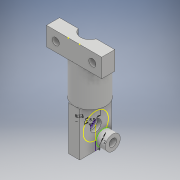
# Autodesk Inventor part: frontChassis
Saved by Autodesk Inventor 2018 (Build 220112000, 112)
## iProperties
Created: 2018-02-04
Part Number: frontChassis
Material: Generic
Document SubType Name: Modeling
Designer: Prakash
Density: 1 g/cm^3
Appearance: Default
Author: Prakash
Autodesk Inventor part; units mm, degrees
ref_plane "YZ Plane" through (0, 0, 0) normal (1, 0, 0) x (0, 1, 0)
ref_plane "XZ Plane" through (0, 0, 0) normal (0, 1, 0) x (-1, 0, 0)
ref_plane "XY Plane" through (0, 0, 0) normal (0, 0, 1) x (1, 0, 0)
sketch "Sketch1" plane through (0, 0, 0) normal (0, 0, 1) x (1, 0, 0)
  line L0 (0, 0) -> (0, 7)
  line L1 (0, 7) -> (10, 7)
  arc A0 (10, 7) -> (19.5394, 7) centre (14.7697, 8.5) ccw
  line L2 (19.5394, 7) -> (29.5394, 7)
  line L3 (29.5394, 7) -> (29.5394, 0)
  line L4 (29.5394, 0) -> (0, 0)
  dimension "d0" = 10
  dimension "d1" = 5
  dimension "d2" = 7
  dimension "d4" = 1.5
  constraints: 10 end point, 3 perpendicular, 2 collinear, 2 point on circle, 1 centre point, 1 horizontal, 1 vertical
  measures "d0" distance of L0.end L1.end
  measures "d1" radius of A0
  measures "d2" distance of L0.start L0.end
  measures "d4" distance from line of L1 A0.centre
extrude "Extrusion1" add sketch "Sketch1" against normal blind 10
sketch "Sketch3" plane through (0, 0, -10) normal (0, 0, -1) x (-1, 0, 0)
  line L0 (0, 0) -> (0, 7) projected
  line L1 (0, 7) -> (-10, 7) projected
  arc A0 (-19.5394, 7) -> (-10, 7) centre (-14.7697, 8.5) ccw projected
  line L2 (-19.5394, 7) -> (-29.5394, 7) projected
  line L3 (-29.5394, 7) -> (-29.5394, 0) projected
  line L4 (-29.5394, 0) -> (0, 0) projected
  circle A1 centre (-14.7697, 8.5) radius 5
  circle A2 centre (-14.7697, 8.5) radius 8.5
  line L5 (-29.5394, 0) -> (0, 0) projected
  constraints: 2 centre point, 1 coincident, 1 concentric, 1 tangent
extrude "Extrusion2" add sketch "Sketch3" along normal blind 20 contours A2 L2 A0 L1 | L1 A1 L2 A2
sketch "Sketch4" plane through (14.7697, 8.5, -30) normal (0, 0, -1) x (-1, 0, 0)
  line L0 (-14.7697, -8.5) -> (14.7697, -8.5) projected
  line L1 (0, -8.5) -> (3, -8.5)
  line L2 (0, -8.5) -> (-3, -8.5)
  circle A0 centre (0, 0) radius 5 projected
  circle A1 centre (0, 0) radius 8.5 projected
  line L3 (-3, -8.5) -> (3, -8.5)
  line L4 (3, -8.5) -> (3, 8.5)
  line L5 (3, 8.5) -> (-3, 8.5)
  line L6 (-3, 8.5) -> (-3, -8.5)
  dimension "d18" = 3
  dimension "d19" = 3
  constraints: 12 end point, 2 parallel, 2 point on line, 1 horizontal, 1 midpoint, 1 perpendicular, 1 tangent
  measures "d18" distance of L1.start L1.end
  measures "d19" distance of L1.start L2.end
extrude "Extrusion3" add sketch "Sketch4" along normal blind 23.5 contours L6 A1 L0 | A1 L4 L0 | A1 L6 A0 L4 | L6 L5 A1 | A1 L4 A0 L6 | L6 A0 L4 | L5 L4 A1
sketch "Sketch6" plane through (11.7697, 4.5, -30) normal (-1, 0, 0) x (0, 0, 1)
  line L0 (0, 12.5) -> (-23.5, 12.5) projected
  line L1 (-11.75, 12.5) -> (-11.75, 4)
  line L2 (-11.75, 4) -> (-23.5, 4)
  circle A0 centre (-11.75, 4) radius 6.75
  circle A1 centre (-11.75, 4) radius 3
  circle A2 centre (-11.75, 4) radius 6
  point P0 (30, -4.5)
  dimension "d26" = 8.5
  dimension "d27" = 13.5
  dimension "d28" = 6
  dimension "d29" = 12
  constraints: 4 end point, 3 centre point, 3 coincident, 1 midpoint, 1 perpendicular, 1 vertical
  measures "d26" distance of L1.start L1.end
  measures "d27" diameter of A0
  measures "d28" diameter of A1
  measures "d29" diameter of A2
extrude "Extrusion4" cut sketch "Sketch6" against normal blind 1 contours A0 L2 A2 L1 | L1 A2 L2 A0
extrude "Extrusion5" cut sketch "Sketch6" against normal blind 4 contours A2 L2 A1 L1 | L1 A1 L2 A2
extrude "Extrusion6" cut sketch "Sketch6" against normal up to surface (6 mm away) contours A1 L2 L1 | L1 L2 A1
sketch "Sketch7" plane through (17.7697, 4.5, -30) normal (1, 0, 0) x (0, 0, -1)
  line L0 (11.75, 4) -> (23.5, 4) projected
  circle A0 centre (11.75, 4) radius 6.75 projected
  line L1 (18.5, 4) -> (23.5, 4)
  circle A1 centre (19.2602, 8.1796) radius 2
  circle A2 centre (19.2602, 8.1796) radius 4
  point P0 (-30, -4.5)
  dimension "d40" = 4
  dimension "d41" = 2
  constraints: 2 centre point, 2 end point, 1 coincident, 1 collinear, 1 horizontal alignment, 1 point on line, 1 other
  measures "d40" diameter of A1
  measures "d41" radial gap between concentric circles of A1 A2
extrude "Extrusion7" add sketch "Sketch7" along normal blind 5 contours A2 A0 A1 | A0 A1 A2
extrude "Extrusion8" cut sketch "Sketch7" against normal blind 2 contours A1 A0 | A0 A1
sketch "Sketch8" plane through (0, 7, 0) normal (0, 1, 0) x (1, 0, 0)
  line L0 (0, 0) -> (10, 0) projected
  line L1 (5, 0) -> (5, 10)
  line L2 (0, 10) -> (6.4031, 10) projected
  line L3 (19.5394, 0) -> (29.5394, 0) projected
  line L4 (24.5394, 0) -> (24.5394, 10)
  point P0 (24.5394, 5)
  point P1 (5, 5)
  constraints: 4 end point, 4 midpoint, 2 vertical, 1 point on line
hole "Hole2" at (5, 7, -5) at (24.5394, 7, -5) direction (0, -1, 0) diameter 3.797 end through all clearance for "Flat Head Machine Screw (82)" size "#6" standard "Ansi Unified Screw Threads"
body "Solid1"
